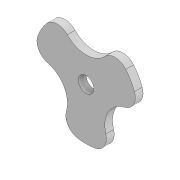
# Autodesk Inventor part: knob
Saved by Autodesk Inventor 2020 (Build 240168000, 168)
## iProperties
Created: 2021-06-15
Part Number: knob
Material: Generic
Document SubType Name: Modeling
Designer: Aidan Lee
Density: 1 g/cm^3
Appearance: Default
Author: Aidan Lee
Autodesk Inventor part; units mm, degrees
ref_plane "YZ Plane" through (0, 0, 0) normal (1, 0, 0) x (0, 1, 0)
ref_plane "XZ Plane" through (0, 0, 0) normal (0, 1, 0) x (-1, 0, 0)
ref_plane "XY Plane" through (0, 0, 0) normal (0, 0, 1) x (1, 0, 0)
sketch "Sketch1" plane through (0, 0, 0) normal (0, 0, 1) x (1, 0, 0)
  circle A0 centre (0, 0) radius 3
  circle A1 centre (0, 0) radius 20
  circle A2 centre (0, 20) radius 10.073
  circle A3 centre (-17.3205, -10) radius 10.073
  circle A4 centre (17.3205, -10) radius 10.073
  arc A5 (-7.2901, 13.0488) -> (-15.3936, 12.7686) centre (-11.2172, 9.3043) ccw
  line L0 (0, 39.6436) -> (0, 33.3002) construction
  arc A6 (15.3936, 12.7686) -> (7.2901, 13.0488) centre (11.2172, 9.3043) ccw
  arc A7 (-7.6556, -12.8378) -> (-3.3611, -19.7156) centre (-2.4492, -14.3665) ccw
  arc A8 (-18.7547, 6.947) -> (-14.9457, -0.211) centre (-13.6664, 5.0622) ccw
  arc A9 (14.9457, -0.211) -> (18.7547, 6.947) centre (13.6664, 5.0622) ccw
  arc A10 (3.3611, -19.7156) -> (7.6556, -12.8378) centre (2.4492, -14.3665) ccw
  line L1 (0, 9.927) -> (-4.2832, 9.927) construction
  point P0 (7.3052, 13.0646)
  point P1 (-13.6431, 13.6431)
  point P2 (-14.9669, -0.2058)
  point P3 (-7.6556, -12.8378)
  point P4 (-13.6431, -13.6431)
  point P5 (7.6617, -12.8588)
  point P6 (14.9457, -0.211)
  point P7 (15.3936, 12.7686)
  point P8 (-3.3611, -19.7156)
  point P9 (3.3611, -19.7156)
  point P10 (18.7547, 6.947)
  dimension "d0" = 6
  dimension "d1" = 40
  dimension "d4" = 360
  dimension "d8" = 360
  constraints: 16 point on circle, 11 centre point, 4 end point, 3 symmetric about line, 3 tangent, 2 coincident, 1 horizontal, 1 vertical, 1 vertical alignment, 33 other
  measures "d0" diameter of A0
  measures "d1" diameter of A1
extrude "Extrusion1" add sketch "Sketch1" along normal blind 3 contours A9 A4 A10 A1 A7 A3 A8 A5 A2 A6
body "Solid1"
